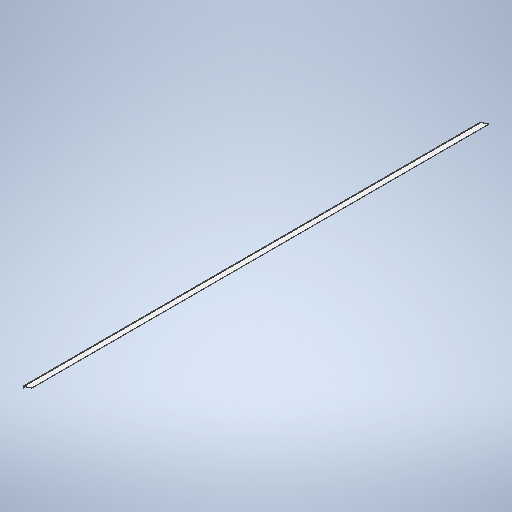
# Autodesk Inventor part: Drip_Edge_For_Back
Saved by Autodesk Inventor 2025.1 (Build 291241020, 241B)
## iProperties
Created: 2024-09-15
Part Number: Drip_Edge_For_Back
Material: Aluminum 6061
Document SubType Name: Modeling
Designer: Tom
Density: 2.7 g/cm^3
Appearance: White
Author: Tom
Autodesk Inventor part; units mm, degrees
ref_plane "YZ Plane" through (0, 0, 0) normal (1, 0, 0) x (0, 1, 0)
ref_plane "XZ Plane" through (0, 0, 0) normal (0, 1, 0) x (-1, 0, 0)
ref_plane "XY Plane" through (0, 0, 0) normal (0, 0, 1) x (1, 0, 0)
sketch "Sketch1" plane through (0, 0, 0) normal (0, 0, 1) x (1, 0, 0)
  line L0 (0, 0) -> (3294.2276, 1099.144)
  line L1 (3294.2276, 1246.4151) -> (-135.0962, 102.1952)
  line L2 (0, 0) -> (-135.0962, 0)
  line L3 (-135.0962, 0) -> (-135.0962, 102.1952)
  line L4 (-135.0962, 102.1952) -> (1627.6312, 690.3426)
  line L5 (3294.2276, 1099.144) -> (3263.9, 1099.144)
  line L6 (3294.2276, 1099.144) -> (3294.2276, 1246.4151)
  line L7 (-88.9, 0) -> (-88.9, 117.6089)
  line L8 (3263.9, 1089.025) -> (3263.9, 1236.2961)
  line L9 (-135.0962, 102.1952) -> (-160.4962, 102.1952)
  line L10 (-160.4962, 102.1952) -> (-160.4962, 0)
  line L11 (-160.4962, 0) -> (-135.0962, 0)
  line L12 (-135.0962, 102.1952) -> (-140.1208, 117.2541)
  line L13 (-140.1208, 117.2541) -> (150.6173, 214.261)
  line L14 (150.6173, 214.261) -> (155.6418, 199.2021)
  line L15 (-27.6261, 154.7888) -> (-28.631, 157.8005)
  line L16 (-28.631, 157.8005) -> (-173.1962, 109.5652)
  line L17 (-173.1962, 109.5652) -> (-163.6712, 101.107)
  line L18 (-163.6712, 101.107) -> (-163.6712, 92.6488)
  line L19 (-163.6712, 92.6488) -> (-173.1962, 86.9102)
  line L20 (-171.5578, 84.1906) -> (-160.4962, 90.855)
  line L21 (-160.4962, 90.855) -> (-160.4962, 102.5338)
  line L22 (-160.4962, 102.5338) -> (-166.9808, 108.292)
  line L23 (-166.9808, 108.292) -> (-27.6261, 154.7888)
  line L24 (-171.5578, 84.1906) -> (-173.1962, 86.9102)
  line L25 (-173.1962, 109.5652) -> (-173.1962, 86.9102)
  point P0 (-160.4962, 90.855)
  point P1 (-160.4962, 101.4128)
  dimension "d5" = 139.7
  dimension "d17" = 88.9
  dimension "d19" = 3352.8
  dimension "d23" = 30.3276
  dimension "d28" = 46.1962
  dimension "d33" = 1089.025
  dimension "d36" = 25.4
  dimension "d37" = 15.875
  dimension "d49" = 3.175
  dimension "d50" = 3.175
  dimension "d51" = 3.175
  dimension "d52" = 3.175
  dimension "d54" = 8.4582
  dimension "d55" = 8.4582
  dimension "d61" = 8.4582
  dimension "d62" = 152.4
  constraints: 52 end point, 7 point on line, 6 parallel, 6 perpendicular, 5 vertical, 3 collinear, 3 horizontal, 2 coincident
  measures "d5" distance between parallel lines of L1 L0
  measures "d17" distance from line of L7 point (0, 0)
  measures "d19" distance between parallel lines of L7 L8
  measures "d23" distance between parallel lines of L6 L8
  measures "d28" distance between parallel lines of L3 L7
  measures "d33" vertical distance of L8.start point (0, 0)
  measures "d36" distance of L10.end L2.end
  measures "d37" distance of L13.end L14.end
  measures "d49" distance between parallel lines of L16 L23
  measures "d50" distance between parallel lines of L18 L21
  measures "d51" distance between parallel lines of L17 L22
  measures "d52" distance between parallel lines of L19 L20
  measures "d54" distance of L18.end L17.end
  measures "d55" vertical distance of L20.start L18.end
  measures "d61" vertical distance of L17.end L16.end
  measures "d62" distance of L15.end L16.end
extrude "Extrusion2" add sketch "Sketch1" along normal blind 7429.8302 contours L10 L20 L24 L19 L18 L17 L16 L15 L13 L23 L22 L21
body "Solid2"
